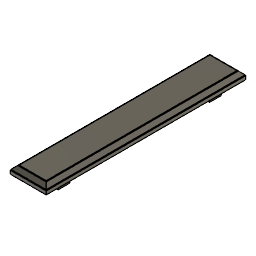
sensor-rod-lid (Autodesk Fusion 360 design; units mm, degrees)
part number: 2026-07-21-14-48-35-226
Autodesk Fusion 360 part; units mm, degrees
sketch "Sketch1" plane through (0, 0, 0) normal (0, 0, 1) x (1, 0, 0)
  line L0 (9, 50) -> (-9, 50)
  line L1 (-9, 50) -> (-9, -50)
  line L2 (-9, -50) -> (9, -50)
  line L3 (9, -50) -> (9, 50)
  line L4 (9, 50) -> (-9, -50) construction
  line L5 (-9, 50) -> (9, -50) construction
  line L6 (-4.925, 41.8706) -> (4.925, 41.8706)
  line L7 (4.925, 41.8706) -> (4.925, 35.9206)
  line L8 (4.925, 35.9206) -> (-4.925, 35.9206)
  line L9 (-4.925, 35.9206) -> (-4.925, 41.8706)
  line L10 (-4.925, 41.8706) -> (4.925, 35.9206) construction
  line L11 (4.925, 41.8706) -> (-4.925, 35.9206) construction
  line L12 (4.925, -33.9994) -> (-4.925, -33.9994)
  line L13 (-4.925, -33.9994) -> (-4.925, -39.9494)
  line L14 (-4.925, -39.9494) -> (4.925, -39.9494)
  line L15 (4.925, -39.9494) -> (4.925, -33.9994)
  line L16 (4.925, -33.9994) -> (-4.925, -39.9494) construction
  line L17 (-4.925, -33.9994) -> (4.925, -39.9494) construction
  point P0 (0, 38.8956)
  point P1 (0, -36.9744)
  dimension "d1" = 18
  dimension "d2" = 100
  dimension "d3" = 5.95
  dimension "d4" = 9.85
  dimension "d5" = 5.95
  dimension "d9" = 4.925
  dimension "d10" = 33.9994
  dimension "d11" = 69.92
  constraint horizontal L0
  constraint perpendicular L0 L1
  constraint parallel L0 L2
  constraint parallel L1 L3
  constraint coincident L4 origin
  constraint coincident L5 origin
  constraint horizontal L6
  constraint perpendicular L6 L7
  constraint parallel L6 L8
  constraint parallel L7 L9
  constraint coincident L10 P0
  constraint coincident L11 P0
  constraint horizontal L12
  constraint perpendicular L12 L13
  constraint parallel L12 L14
  constraint parallel L13 L15
  constraint coincident L16 P1
  constraint coincident L17 P1
  constraint collinear origin P0 P1
  constraint collinear L7 L15
  constraint collinear L9 L13
  measures "d1" distance of L1.end L2.end
  measures "d2" distance of L0.end L1.end
  measures "d3" distance of L6.end L7.end
  measures "d4" distance of L13.end L14.end
  measures "d5" distance of L12.end L13.end
  measures "d9" distance of origin L15
  measures "d10" distance of origin L12
  measures "d11" distance of L8 L12
extrude "Extrude1" add sketch "Sketch1" against normal blind 4.85 contours L6 L7 L8 L9 | L12 L13 L14 L15 makes body 1 at (-1.6417, 37.9039, 0) makes body 2 at (1.6417, -35.9827, 0)
sketch "Sketch2" plane through (0, 0, 0) normal (0, 0, 1) x (1, 0, 0)
  line L0 (9, 50) -> (-9, 50)
  line L1 (-9, 50) -> (-9, -50)
  line L2 (-9, -50) -> (9, -50)
  line L3 (9, -50) -> (9, 50)
  line L4 (9, 50) -> (-9, -50) construction
  line L5 (-9, 50) -> (9, -50) construction
  dimension "d14" = 18
  dimension "d15" = 100
  constraint horizontal L0
  constraint perpendicular L0 L1
  constraint parallel L0 L2
  constraint parallel L1 L3
  constraint coincident L4 origin
  constraint coincident L5 origin
  measures "d14" distance of L1.end L2.end
  measures "d15" distance of L0.end L1.end
extrude "Extrude2" add sketch "Sketch2" along normal blind 4 bodies 1 2
chamfer "Chamfer1" distance 2 angle 45 1 faces at (-3, -16.6667, 4) on bodies 1
fillet "Fillet1" radius 0.5 8 edges at (-7, 0, 4) (0, -48, 4) (7, 0, 4) (0, 48, 4) (-9, 0, 2) (0, -50, 2) (0, 50, 2) (9, 0, 2) on bodies 1
